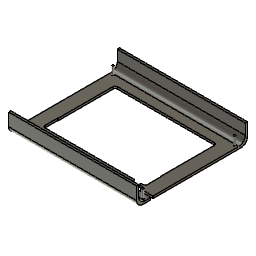
MUS3005Top (Autodesk Fusion 360 design; units mm, degrees)
Autodesk Fusion 360 part; units mm, degrees
sketch "Sketch1" plane through (0, 0, 0) normal (0, 0, 1) x (1, 0, 0)
  line L0 (0, 0) -> (300, 0)
  line L1 (300, 0) -> (300, 260)
  line L2 (300, 260) -> (0, 260)
  line L3 (0, 260) -> (0, 0)
  circle A0 centre (7.5, 22.5) radius 2.25
  circle A1 centre (292.5, 22.5) radius 2.25
  circle A2 centre (7.5, 237.5) radius 2.25
  circle A3 centre (292.5, 237.5) radius 2.25
  dimension "d1" = 300
  dimension "d2" = 260
  dimension "d3" = 4.5
  dimension "d4" = 4.5
  dimension "d5" = 4.5
  dimension "d6" = 4.5
  dimension "d7" = 22.5
  dimension "d8" = 7.5
  dimension "d9" = 22.5
  dimension "d10" = 7.5
  dimension "d11" = 7.5
  dimension "d12" = 22.5
  dimension "d13" = 22.5
  dimension "d14" = 7.5
  constraint horizontal L0
  constraint vertical L1
  constraint horizontal L2
  constraint vertical L3
  constraint coincident L0.start L3.end
  measures "d1" distance of L0.start L0.end
  measures "d2" distance of L0.start L2.end
  measures "d3" diameter of A0
  measures "d4" diameter of A1
  measures "d5" diameter of A2
  measures "d6" diameter of A3
  measures "d7" distance of L0 A0.centre
  measures "d8" distance of L3 A0.centre
  measures "d9" distance of L0 A1.centre
  measures "d10" distance of L1 A1.centre
  measures "d11" distance of L3 A2.centre
  measures "d12" distance of L2 A2.centre
  measures "d13" distance of L2 A3.centre
  measures "d14" distance of L1 A3.centre
extrude "Extrude1" add sketch "Sketch1" along normal blind 5
extrude "Extrude2" add sketch "Sketch1" along normal blind 25 contours A0
extrude "Extrude3" add sketch "Sketch1" along normal blind 25 contours A2
extrude "Extrude4" add sketch "Sketch1" along normal blind 25 contours A3
extrude "Extrude5" add sketch "Sketch1" along normal blind 25 contours A1
sketch "Sketch2" plane through (0, 0, 5) normal (0, 0, 1) x (-1, 0, 0)
  circle A0 centre (-7.5, -22.5) radius 2.25
  circle A1 centre (-7.5, -237.5) radius 2.25
  circle A2 centre (-292.5, -22.5) radius 2.25
  circle A3 centre (-292.5, -237.5) radius 2.25
  line L0 (0, -260) -> (0, 0)
  line L1 (0, 0) -> (-300, 0)
  line L2 (-300, 0) -> (-300, -260)
  line L3 (-300, -260) -> (0, -260)
  line L4 (-30, -220) -> (-270, -220)
  line L5 (-270, -220) -> (-270, -55.5)
  line L6 (-270, -50.5) -> (-30, -50.5)
  line L7 (-30, -50.5) -> (-30, -220)
  line L8 (-300, -260) -> (0, -260)
  line L9 (0, 0) -> (-300, 0)
  line L10 (0, -260) -> (0, 0)
  line L11 (-300, 0) -> (-300, -260)
  line L12 (-30, -220) -> (-270, -220)
  line L13 (-270, -220) -> (-270, -219)
  line L14 (-270, -219) -> (-30, -219)
  line L15 (-30, -219) -> (-30, -220)
  line L16 (-270, -220) -> (-269, -220)
  line L17 (-269, -220) -> (-269, -85)
  line L18 (-269, -85) -> (-270, -85)
  line L19 (-270, -85) -> (-270, -220)
  line L20 (-30, -220) -> (-31, -220)
  line L21 (-31, -220) -> (-31, -85)
  line L22 (-31, -85) -> (-30, -85)
  line L23 (-30, -85) -> (-30, -220)
  line L24 (-36, -219) -> (-36, -219)
  line L25 (-36, -219) -> (-36, -214)
  line L26 (-36, -214) -> (-31, -214)
  line L27 (-31, -214) -> (-31, -214)
  arc A4 (-36, -219) -> (-31, -214) centre (-36, -214) ccw
  line L28 (-264, -219) -> (-264, -219)
  line L29 (-264, -219) -> (-264, -214)
  line L30 (-264, -214) -> (-269, -214)
  line L31 (-269, -214) -> (-269, -214)
  arc A5 (-269, -214) -> (-264, -219) centre (-264, -214) ccw
  line L32 (-265, -50.5) -> (-265, -50.5)
  line L33 (-265, -50.5) -> (-265, -55.5)
  line L34 (-265, -55.5) -> (-270, -55.5)
  line L35 (-270, -55.5) -> (-270, -50.5)
  arc A6 (-265, -50.5) -> (-270, -55.5) centre (-265, -55.5) ccw
  line L36 (-35, -50.5) -> (-35, -50.5)
  line L37 (-35, -50.5) -> (-35, -55.5)
  line L38 (-35, -55.5) -> (-30, -55.5)
  line L39 (-30, -55.5) -> (-30, -55.5)
  arc A7 (-30, -55.5) -> (-35, -50.5) centre (-35, -55.5) ccw
  point P0 (-31, -219)
  point P1 (-269, -219)
  dimension "d25" = 240
  dimension "d26" = 169.5
  dimension "d27" = 40
  dimension "d28" = 50.5
  dimension "d29" = 30
  dimension "d30" = 30
  dimension "d31" = 1
  dimension "d32" = 135
  dimension "d33" = 1
  dimension "d34" = 135
  dimension "d35" = 1
  dimension "d36" = 5
  dimension "d37" = 5
  dimension "d38" = 5
  dimension "d39" = 5
  dimension "d40" = 5
  dimension "d41" = 5
  dimension "d42" = 5
  dimension "d43" = 5
  dimension "d44" = 5
  dimension "d45" = 5
  dimension "d46" = 5
  dimension "d47" = 5
  constraint horizontal L4
  constraint vertical L5
  constraint horizontal L6
  constraint vertical L7
  constraint horizontal L12
  constraint vertical L13
  constraint horizontal L14
  constraint vertical L15
  constraint horizontal L16
  constraint vertical L17
  constraint horizontal L18
  constraint vertical L19
  constraint horizontal L20
  constraint vertical L21
  constraint horizontal L22
  constraint vertical L23
  constraint vertical L25
  constraint horizontal L26
  constraint coincident L21 P0
  constraint coincident L14 P0
  constraint coincident P0 L24
  constraint coincident P0 L27
  constraint vertical L29
  constraint horizontal L30
  constraint coincident L14 P1
  constraint coincident L17 P1
  constraint coincident P1 L28
  constraint coincident P1 L31
  constraint vertical L33
  constraint horizontal L34
  constraint vertical L35
  constraint coincident L6.start L32
  constraint coincident L6.start L5
  constraint tangent L5 A6
  constraint vertical L37
  constraint horizontal L38
  constraint coincident L6.end L39
  constraint coincident L6.end L36
  measures "d25" distance of L4.start L4.end
  measures "d26" distance of L4.start L6.end
  measures "d27" distance of L4 L8
  measures "d28" distance of L6 L9
  measures "d29" distance of L7 L10
  measures "d30" distance of L5 L11
  measures "d31" distance of L4.end L13.end
  measures "d32" distance of L20.end L21.end
  measures "d33" distance of L4.start L20.end
  measures "d34" distance of L16.end L17.end
  measures "d35" distance of L17.end L18.end
  measures "d36" distance of P0 L24.start
  measures "d37" distance of L24.start L25.end
  measures "d38" radius of A4
  measures "d39" distance of P1 L28.start
  measures "d40" distance of L28.start L29.end
  measures "d41" radius of A5
  measures "d42" distance of L6.start L32.start
  measures "d43" distance of L32.start L33.end
  measures "d44" radius of A6
  measures "d45" distance of L6.end L36.start
  measures "d46" distance of L36.start L37.end
  measures "d47" radius of A7
extrude "Extrude6" cut sketch "Sketch2" against normal blind 5 contours L5 L6 L7 L14 L17 L18 L21 L22 L25 L26 L29 L30 L33 L34 L37 L38
extrude "Extrude7" cut sketch "Sketch2" against normal blind 5 contours L37 L38 A7
extrude "Extrude8" cut sketch "Sketch2" against normal blind 5 contours L33 L34 A6
extrude "Extrude9" cut sketch "Sketch2" against normal blind 5 contours L29 L30 A5
extrude "Extrude10" cut sketch "Sketch2" against normal blind 5 contours L25 L26 A4
sketch "Sketch3" plane through (0, 0, 5) normal (0, 0, 1) x (-1, 0, 0)
  arc A0 (-36, -219) -> (-31, -214) centre (-36, -214) ccw
  line L0 (-36, -219) -> (-264, -219)
  arc A1 (-269, -214) -> (-264, -219) centre (-264, -214) ccw
  line L1 (-269, -214) -> (-269, -85)
  line L2 (-269, -85) -> (-270, -85)
  line L3 (-270, -85) -> (-270, -55.5)
  arc A2 (-265, -50.5) -> (-270, -55.5) centre (-265, -55.5) ccw
  line L4 (-265, -50.5) -> (-35, -50.5)
  arc A3 (-30, -55.5) -> (-35, -50.5) centre (-35, -55.5) ccw
  line L5 (-30, -55.5) -> (-30, -85)
  line L6 (-30, -85) -> (-31, -85)
  line L7 (-31, -85) -> (-31, -214)
  line L8 (0, -260) -> (0, 0)
  line L9 (0, 0) -> (-300, 0)
  line L10 (-300, 0) -> (-300, -260)
  line L11 (-300, -260) -> (0, -260)
  circle A4 centre (-292.5, -237.5) radius 2.25
  circle A5 centre (-292.5, -22.5) radius 2.25
  circle A6 centre (-7.5, -237.5) radius 2.25
  circle A7 centre (-7.5, -22.5) radius 2.25
  line L12 (0, 0) -> (-300, 0)
  line L13 (-300, 0) -> (-300, -5)
  line L14 (-300, -5) -> (0, -5)
  line L15 (0, -5) -> (0, 0)
  line L16 (0, -260) -> (-300, -260)
  line L17 (-300, -260) -> (-300, -255)
  line L18 (-300, -255) -> (0, -255)
  line L19 (0, -255) -> (0, -260)
  dimension "d58" = 300
  dimension "d59" = 5
  dimension "d60" = 300
  dimension "d61" = 5
  constraint horizontal L12
  constraint vertical L13
  constraint horizontal L14
  constraint vertical L15
  constraint coincident L8.end L9.start
  constraint horizontal L16
  constraint vertical L17
  constraint horizontal L18
  constraint vertical L19
  constraint coincident L8.start L11.end
  measures "d58" distance of L8.end L9.end
  measures "d59" distance of L8.end L14.end
  measures "d60" distance of L8.start L10.end
  measures "d61" distance of L8.start L18.end
extrude "Extrude11" add sketch "Sketch3" along normal blind 40 contours L8 L10 L11 L16 L17 L18 L19
extrude "Extrude12" add sketch "Sketch3" along normal blind 40 contours L8 L9 L10 L12 L13 L14 L15
fillet "Fillet1" radius 15 1 edges at (150, 255, 5)
fillet "Fillet2" radius 15 1 edges at (150, 260, 0)
fillet "Fillet3" radius 15 1 edges at (150, 5, 5)
fillet "Fillet4" radius 15 1 edges at (150, 0, 0)
sketch "Sketch4" plane through (0, 0, 0) normal (0, 0, -1) x (1, 0, 0)
  line L0 (300, -15) -> (0, -15)
  line L1 (0, -15) -> (0, -245)
  line L2 (0, -245) -> (300, -245)
  line L3 (300, -245) -> (300, -15)
  arc A0 (31, -214) -> (36, -219) centre (36, -214) ccw
  line L4 (31, -214) -> (31, -85)
  line L5 (31, -85) -> (30, -85)
  line L6 (30, -85) -> (30, -55.5)
  arc A1 (35, -50.5) -> (30, -55.5) centre (35, -55.5) ccw
  line L7 (35, -50.5) -> (265, -50.5)
  arc A2 (270, -55.5) -> (265, -50.5) centre (265, -55.5) ccw
  line L8 (270, -55.5) -> (270, -85)
  line L9 (270, -85) -> (269, -85)
  line L10 (269, -85) -> (269, -214)
  arc A3 (264, -219) -> (269, -214) centre (264, -214) ccw
  line L11 (264, -219) -> (36, -219)
  line L12 (245, -50.5) -> (260, -50.5)
  line L13 (260, -50.5) -> (260, -33.5)
  line L14 (260, -33.5) -> (245, -33.5)
  line L15 (245, -33.5) -> (245, -50.5)
  line L16 (260, -33.5) -> (270, -33.5)
  line L17 (270, -33.5) -> (270, -45.5)
  line L18 (270, -45.5) -> (260, -45.5)
  line L19 (260, -45.5) -> (260, -33.5)
  line L20 (270, -33.5) -> (300, -33.5)
  line L21 (300, -33.5) -> (300, -38.5)
  line L22 (300, -38.5) -> (270, -38.5)
  line L23 (270, -38.5) -> (270, -33.5)
  dimension "d74" = 15
  dimension "d75" = 17
  dimension "d76" = 10
  dimension "d77" = 12
  dimension "d78" = 30
  dimension "d79" = 30
  dimension "d80" = 5
  constraint horizontal L12
  constraint vertical L13
  constraint horizontal L14
  constraint vertical L15
  constraint coincident L7 L12.start
  constraint horizontal L16
  constraint vertical L17
  constraint horizontal L18
  constraint vertical L19
  constraint horizontal L20
  constraint vertical L21
  constraint horizontal L22
  constraint vertical L23
  measures "d74" distance of L12.start L12.end
  measures "d75" distance of L12.start L14.end
  measures "d76" distance of L13.end L16.end
  measures "d77" distance of L16.end L17.end
  measures "d78" distance of L3 L17
  measures "d79" distance of L16.end L20.end
  measures "d80" distance of L16.end L22.end
extrude "Extrude13" cut sketch "Sketch4" against normal blind 5 contours L7 L12 L13 L14 L15 L19
extrude "Extrude14" cut sketch "Sketch4" against normal blind 5 contours L13 L16 L17 L18 L19 L23
extrude "Extrude15" cut sketch "Sketch4" against normal blind 5 contours L3 L17 L20 L21 L22 L23
fillet "Fillet5" radius 1 1 edges at (245, 50.5, 2.5)
fillet "Fillet6" radius 1 1 edges at (245, 33.5, 2.5)
fillet "Fillet7" radius 1 1 edges at (260, 50.5, 2.5)
fillet "Fillet8" radius 1 1 edges at (260, 45.5, 2.5)
fillet "Fillet9" radius 1 1 edges at (270, 45.5, 2.5)
fillet "Fillet10" radius 1 1 edges at (270, 38.5, 2.5)
fillet "Fillet11" radius 1 1 edges at (300, 33.5, 2.5)
fillet "Fillet12" radius 1 1 edges at (300, 38.5, 2.5)
sketch "Sketch5" plane through (0, 0, 0) normal (0, 0, -1) x (1, 0, 0)
  arc A0 (300, -39.5) -> (299, -38.5) centre (299, -39.5) ccw
  line L0 (299, -38.5) -> (271, -38.5)
  arc A1 (271, -38.5) -> (270, -39.5) centre (271, -39.5) ccw
  line L1 (270, -39.5) -> (270, -44.5)
  arc A2 (269, -45.5) -> (270, -44.5) centre (269, -44.5) ccw
  line L2 (269, -45.5) -> (261, -45.5)
  arc A3 (261, -45.5) -> (260, -46.5) centre (261, -46.5) ccw
  line L3 (260, -46.5) -> (260, -49.5)
  arc A4 (260, -49.5) -> (261, -50.5) centre (261, -49.5) ccw
  line L4 (261, -50.5) -> (265, -50.5)
  arc A5 (270, -55.5) -> (265, -50.5) centre (265, -55.5) ccw
  line L5 (270, -55.5) -> (270, -85)
  line L6 (270, -85) -> (269, -85)
  line L7 (269, -85) -> (269, -214)
  arc A6 (264, -219) -> (269, -214) centre (264, -214) ccw
  line L8 (264, -219) -> (36, -219)
  arc A7 (31, -214) -> (36, -219) centre (36, -214) ccw
  line L9 (31, -214) -> (31, -85)
  line L10 (31, -85) -> (30, -85)
  line L11 (30, -85) -> (30, -55.5)
  arc A8 (35, -50.5) -> (30, -55.5) centre (35, -55.5) ccw
  line L12 (35, -50.5) -> (244, -50.5)
  arc A9 (244, -50.5) -> (245, -49.5) centre (244, -49.5) ccw
  line L13 (245, -49.5) -> (245, -34.5)
  arc A10 (246, -33.5) -> (245, -34.5) centre (246, -34.5) ccw
  line L14 (246, -33.5) -> (299, -33.5)
  arc A11 (299, -33.5) -> (300, -32.5) centre (299, -32.5) ccw
  line L15 (300, -32.5) -> (300, -15)
  line L16 (300, -15) -> (0, -15)
  line L17 (0, -15) -> (0, -245)
  line L18 (0, -245) -> (300, -245)
  line L19 (300, -245) -> (300, -39.5)
  line L20 (30, -23.5) -> (118, -23.5)
  line L21 (118, -23.5) -> (118, -35.5)
  line L22 (118, -35.5) -> (30, -35.5)
  line L23 (30, -35.5) -> (30, -23.5)
  line L24 (37.5, -27.5) -> (110.5, -27.5)
  line L25 (110.5, -27.5) -> (110.5, -31.5)
  line L26 (110.5, -31.5) -> (37.5, -31.5)
  line L27 (37.5, -31.5) -> (37.5, -27.5)
  circle A12 centre (114.25, -29.5) radius 1.95
  circle A13 centre (33.75, -29.5) radius 1.95
  dimension "d103" = 88
  dimension "d104" = 12
  dimension "d105" = 15
  dimension "d106" = 30
  dimension "d107" = 73
  dimension "d108" = 4
  dimension "d109" = 4
  dimension "d110" = 7.5
  dimension "d111" = 3.9
  dimension "d112" = 3.75
  dimension "d113" = 3.9
  dimension "d114" = 3.75
  dimension "d115" = 6
  dimension "d116" = 6
  constraint horizontal L20
  constraint vertical L21
  constraint horizontal L22
  constraint vertical L23
  constraint horizontal L24
  constraint vertical L25
  constraint horizontal L26
  constraint vertical L27
  measures "d103" distance of L20.start L20.end
  measures "d104" distance of L20.end L21.end
  measures "d105" distance of L12 L22
  measures "d106" distance of L17 L23
  measures "d107" distance of L24.start L24.end
  measures "d108" distance of L24.end L25.end
  measures "d109" distance of L20 L24
  measures "d110" distance of L21 L25
  measures "d111" diameter of A12
  measures "d112" distance of L21 A12.centre
  measures "d113" diameter of A13
  measures "d114" distance of L23 A13.centre
  measures "d115" distance of L22 A13.centre
  measures "d116" distance of L22 A12.centre
extrude "Extrude16" cut sketch "Sketch5" against normal blind 5 contours L24 L25 L26 L27
extrude "Extrude17" cut sketch "Sketch5" against normal blind 5 contours A13
extrude "Extrude18" cut sketch "Sketch5" against normal blind 5 contours A12
